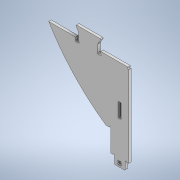
# Autodesk Inventor part: Support A - V2
Saved by Autodesk Inventor 2020 (Build 240168000, 168)
## iProperties
Created: 2020-07-22
Part Number: Support A - V2
Material: Generic
Document SubType Name: Modeling
Designer: Dan Wikman
Density: 1 g/cm^3
Appearance: Default
Author: Dan Wikman
Autodesk Inventor part; units mm, degrees
ref_plane "YZ Plane" through (0, 0, 0) normal (1, 0, 0) x (0, 1, 0)
ref_plane "XZ Plane" through (0, 0, 0) normal (0, 1, 0) x (-1, 0, 0)
ref_plane "XY Plane" through (0, 0, 0) normal (0, 0, 1) x (1, 0, 0)
sketch "Sketch1" plane through (0, 0, 0) normal (0, 0, 1) x (1, 0, 0)
  arc A0 (0, 550) -> (-200, 512.3475) centre (0, 0) ccw construction
  line L0 (-472.3938, -281.6809) -> (-252.3938, -281.6809) construction
  line L1 (-489.0365, 251.6809) -> (-252.3938, 251.6809) construction
  line L2 (-150, 323.3356) -> (-150, 512.3475) construction
  line L3 (-472.3938, 281.6809) -> (-252.3938, 281.6809) construction
  line L4 (-472.3938, -251.6809) -> (-252.3938, -251.6809) construction
  line L5 (-356.435, 15) -> (-576.435, 15) construction
  line L6 (-472.3938, -281.6809) -> (-472.3938, -251.6809) construction
  line L7 (-252.3938, -281.6809) -> (-252.3938, -251.6809) construction
  line L8 (-252.3938, 281.6809) -> (-252.3938, 251.6809) construction
  line L9 (-472.3938, 281.6809) -> (-472.3938, 251.6809) construction
  line L10 (-356.435, 15) -> (-356.435, -15) construction
  line L11 (-356.435, -15) -> (-576.435, -15) construction
  line L12 (-576.435, -15) -> (-576.435, 15) construction
  arc A1 (0, 356.435) -> (-150, 323.3356) centre (0, 0) ccw construction
  arc A2 (-250, -323.3356) -> (-100, -356.435) centre (-100, 0) ccw construction
  arc A3 (-256.5, -512.3475) -> (-260, -512.3475) centre (-258.25, -512.3475) ccw
  line L13 (-278.75, -519.0975) -> (-275, -519.0975)
  line L14 (-278.75, -529.0975) -> (-275, -529.0975)
  line L15 (-275, -519.0975) -> (-275, -529.0975)
  arc A4 (-278.75, -519.0975) -> (-278.75, -522.5975) centre (-278.75, -520.8475) ccw
  arc A5 (-278.75, -525.5975) -> (-278.75, -529.0975) centre (-278.75, -527.3475) ccw
  line L16 (-271.25, -519.0975) -> (-275, -519.0975)
  line L17 (-271.25, -529.0975) -> (-275, -529.0975)
  arc A6 (-271.25, -522.5975) -> (-271.25, -519.0975) centre (-271.25, -520.8475) ccw
  arc A7 (-271.25, -529.0975) -> (-271.25, -525.5975) centre (-271.25, -527.3475) ccw
  line L18 (-356.1192, -15) -> (-549.7954, -15) construction
  line L19 (-252.3938, 251.6809) -> (-489.0365, 251.6809) construction
  arc A8 (-192.6667, 512.3475) -> (-190, 512.3475) centre (-191.3333, 512.3475) ccw construction
  line L20 (-157.3333, 512.3475) -> (-150, 512.3475) construction
  line L21 (-192.6667, 512.3475) -> (-200, 512.3475) construction
  arc A9 (-160, 512.3475) -> (-157.3333, 512.3475) centre (-158.6667, 512.3475) ccw construction
  line L22 (-171.25, 517.8475) -> (-175, 517.8475) construction
  line L23 (-171.25, 520.5142) -> (-171.25, 525.1809) construction
  line L24 (-161.3333, 532.3475) -> (-188.6667, 532.3475) construction
  line L25 (-190, 531.0142) -> (-190, 512.3475) construction
  line L26 (-160, 531.0142) -> (-160, 512.3475) construction
  arc A10 (-160, 531.0142) -> (-161.3333, 532.3475) centre (-161.3333, 531.0142) ccw construction
  arc A11 (-188.6667, 532.3475) -> (-190, 531.0142) centre (-188.6667, 531.0142) ccw construction
  line L27 (-171.25, 527.8475) -> (-175, 527.8475) construction
  line L28 (-175, 532.3475) -> (-175, 535.9358) construction
  line L29 (-175, 517.8475) -> (-175, 527.8475) construction
  arc A12 (-171.25, 517.8475) -> (-171.25, 520.5142) centre (-171.25, 519.1809) ccw construction
  arc A13 (-171.25, 525.1809) -> (-171.25, 527.8475) centre (-171.25, 526.5142) ccw construction
  line L30 (-178.75, 517.8475) -> (-175, 517.8475) construction
  arc A14 (-178.75, 520.5142) -> (-178.75, 517.8475) centre (-178.75, 519.1809) ccw construction
  line L31 (-178.75, 520.5142) -> (-178.75, 525.1809) construction
  arc A15 (-178.75, 527.8475) -> (-178.75, 525.1809) centre (-178.75, 526.5142) ccw construction
  line L32 (-178.75, 527.8475) -> (-175, 527.8475) construction
  arc A16 (-334.9122, -265.623) -> (-335.582, -268.123) centre (-330.582, -268.123) ccw
  line L33 (-328.3782, -254.3059) -> (-334.9122, -265.623)
  arc A17 (-328.3782, -254.3059) -> (-329.8938, -251.6809) centre (-329.8938, -253.4309) ccw
  line L34 (-329.8938, -251.6809) -> (-394.8938, -251.6809)
  line L35 (-362.3938, -251.6809) -> (-362.3938, -293.6041)
  arc A18 (-389.2055, -268.123) -> (-389.8754, -265.623) centre (-394.2055, -268.123) ccw
  arc A19 (-394.8938, -251.6809) -> (-396.4093, -254.3059) centre (-394.8938, -253.4309) ccw
  line L36 (-396.4093, -254.3059) -> (-389.8754, -265.623)
  arc A20 (-389.2055, -291.6809) -> (-389.2055, -288.1809) centre (-389.2055, -289.9309) ccw
  line L37 (-389.2055, -291.6809) -> (-396.7055, -291.6809)
  line L38 (-396.7055, -281.6809) -> (-472.3938, -281.6809)
  line L39 (-328.082, -281.6809) -> (-252.3938, -281.6809)
  arc A21 (-150, 323.3356) -> (-252.3938, -251.6809) centre (0, 0) ccw construction
  arc A22 (-200, 512.3475) -> (-472.3938, -281.6809) centre (0, 0) ccw construction
  line L40 (-271.25, -415.2642) -> (-271.25, -378.7642)
  line L41 (-278.75, -415.2642) -> (-278.75, -378.7642)
  line L42 (-277, -417.0142) -> (-273, -417.0142)
  line L43 (-277, -377.0142) -> (-273, -377.0142)
  arc A23 (-277, -377.0142) -> (-278.75, -378.7642) centre (-277, -378.7642) ccw
  arc A24 (-278.75, -415.2642) -> (-277, -417.0142) centre (-277, -415.2642) ccw
  arc A25 (-273, -417.0142) -> (-271.25, -415.2642) centre (-273, -415.2642) ccw
  arc A26 (-271.25, -378.7642) -> (-273, -377.0142) centre (-273, -378.7642) ccw
  line L44 (-260, -512.3475) -> (-260, -532.5975)
  line L45 (-261.75, -534.3475) -> (-288.25, -534.3475)
  line L46 (-271.25, -522.5975) -> (-271.25, -525.5975)
  line L47 (-278.75, -522.5975) -> (-278.75, -525.5975)
  arc A27 (-290, -532.5975) -> (-288.25, -534.3475) centre (-288.25, -532.5975) ccw
  arc A28 (-261.75, -534.3475) -> (-260, -532.5975) centre (-261.75, -532.5975) ccw
  line L48 (-256.5, -512.3475) -> (-250, -512.3475)
  arc A29 (-396.7055, -288.1809) -> (-396.7055, -291.6809) centre (-396.7055, -289.9309) ccw
  line L49 (-396.7055, -281.6809) -> (-396.7055, -288.1809)
  line L50 (-389.2055, -288.1809) -> (-389.2055, -268.123)
  arc A30 (-335.582, -288.1809) -> (-335.582, -291.6809) centre (-335.582, -289.9309) ccw
  line L51 (-335.582, -291.6809) -> (-328.082, -291.6809)
  arc A31 (-328.082, -291.6809) -> (-328.082, -288.1809) centre (-328.082, -289.9309) ccw
  line L52 (-328.082, -281.6809) -> (-328.082, -288.1809)
  line L53 (-335.582, -288.1809) -> (-335.582, -268.123)
  arc A32 (-252.3938, -283.8475) -> (-252.3938, -287.3475) centre (-252.3938, -285.5975) ccw
  line L54 (-252.3938, -283.8475) -> (-252.3938, -281.6809)
  line L55 (-260, -549.9217) -> (-260, -576.1723)
  line L56 (-160, -561.8521) -> (-260, -561.8521)
  arc A33 (-472.3938, -281.6809) -> (-313.5, -451.9046) centre (0, 0) ccw
  line L57 (-250, -287.3475) -> (-252.3938, -287.3475)
  line L58 (-250, -512.3475) -> (-250, -287.3475)
  arc A34 (-290, -512.3475) -> (-293.5, -512.3475) centre (-291.75, -512.3475) ccw
  line L59 (-293.5, -512.3475) -> (-300, -512.3475)
  line L60 (-300, -512.3475) -> (-300, -451.9046)
  arc A35 (-300, -451.9046) -> (-303.5, -451.9046) centre (-301.75, -451.9046) ccw
  line L61 (-313.5, -451.9046) -> (-303.5, -451.9046)
  line L62 (-290, -532.5975) -> (-290, -512.3475)
  point P0 (0, 512.3475)
  point P1 (0, -512.3475)
  point P2 (-290, -534.3475)
  point P3 (-260, -534.3475)
  point P4 (-59.9119, -534.1417)
  point P5 (-160, 532.3475)
  point P6 (-190, 532.3475)
  point P7 (-389.2055, -259.0142)
  dimension "d13" = 550
  dimension "d17" = 200
  dimension "d18" = 0
  dimension "d54" = 220
  dimension "d56" = 220
  dimension "d57" = 30
  dimension "d59" = 30
  dimension "d62" = 252.3938
  dimension "d73" = 236.6809
  dimension "d74" = 236.6809
  dimension "d75" = 576.435
  dimension "d76" = 472.3938
  dimension "d77" = 472.3938
  dimension "d78" = 30
  dimension "d81" = 220
  dimension "d82" = 252.3938
  dimension "d85" = 356.435
  dimension "d88" = 3.5
  dimension "d89" = 30
  dimension "d90" = 22
  dimension "d103" = 3.75
  dimension "d104" = 3.75
  dimension "d105" = 2.6667
  dimension "d106" = 30
  dimension "d107" = 20
  dimension "d108" = 2.6667
  dimension "d109" = 1.3333
  dimension "d110" = 7.3333
  dimension "d111" = 7.3333
  dimension "d112" = 7.5
  dimension "d113" = 3.75
  dimension "d114" = 3.75
  dimension "d134" = 3.5
  dimension "d135" = 65
  dimension "d136" = 65
  dimension "d137" = 7.3333
  dimension "d138" = 60
  dimension "d139" = 5
  dimension "d140" = 7.5
  dimension "d148" = 1.75
  dimension "d151" = 40
  dimension "d159" = 1.75
  dimension "d160" = 1.75
  dimension "d161" = 1.75
  dimension "d164" = 7.5
  dimension "d170" = 30
  dimension "d171" = 1.75
  dimension "d172" = 10
  dimension "d173" = 3.5
  dimension "d176" = 77.5
  dimension "d180" = 260
  dimension "d182" = 95.3333
  dimension "d184" = 230.6667
  dimension "d185" = 95.3333
  dimension "d186" = 97.0833
  dimension "d187" = 3.5
  constraints: 126 end point, 76 point on circle, 36 centre point, 28 symmetric about line, 16 tangent, 12 vertical, 10 horizontal, 10 perpendicular, 9 point on line, 4 equal radius, 2 collinear, 2 midpoint, 2 parallel, 1 coincident, 10 other
  measures "d13" radius of A0
  measures "d17" distance of point (0, 512.348) A0.end
  measures "d18" horizontal distance of point (0, 0) point (0, 512.348)
  measures "d54" distance of L5.start L5.end
  measures "d56" distance of L0.start L0.end
  measures "d57" distance of L0.end L4.end
  measures "d59" distance between parallel lines of L3 L1
  measures "d62" distance from line of point (0, 0) L7
  measures "d73" distance between parallel lines of L4 L11
  measures "d74" distance between parallel lines of L1 L5
  measures "d75" distance from line of L12 point (0, 0)
  measures "d76" distance from line of point (0, 0) L6
  measures "d77" distance from line of point (0, 0) L9
  measures "d78" distance of L5.start L10.end
  measures "d81" distance between parallel lines of L8 L9
  measures "d82" distance from line of point (0, 0) L8
  measures "d85" distance from line of A0.centre L10
  measures "d88" diameter of A3
  measures "d89" distance of point (-290, -534.348) point (-260, -534.348)
  measures "d90" distance of point (-260, -534.348) L44.start
  measures "d103" distance of L13.start L13.end
  measures "d104" distance of L14.start L14.end
  measures "d105" diameter of A8
  measures "d106" distance of point (-160, 532.348) point (-190, 532.348)
  measures "d107" distance of point (-190, 532.348) L25.end
  measures "d108" diameter of A9
  measures "d109" radius of A10
  measures "d110" distance of L20.start L20.end
  measures "d111" distance of L21.start L21.end
  measures "d112" diameter of L23 L29
  measures "d113" distance of L22.start L22.end
  measures "d114" distance of L27.start L27.end
  measures "d134" diameter of A17
  measures "d135" distance of L34.start L34.end
  measures "d136" distance between centres of A17 A19
  measures "d137" distance from line of point (-389.206, -259.014) L34
  measures "d138" angle of L34 L36
  measures "d139" radius of A18
  measures "d140" distance of L37.start L37.end
  measures "d148" radius of A23
  measures "d151" distance between parallel lines of L42 L43
  measures "d159" radius of A4
  measures "d160" radius of A7
  measures "d161" radius of A27
  measures "d164" distance between parallel lines of L41 L40
  measures "d170" distance between parallel lines of L39 L34
  measures "d171" radius of A20
  measures "d172" distance between parallel lines of L38 L37
  measures "d173" diameter of A32
  measures "d176" horizontal distance of L0.start L34.end
  measures "d180" distance from line of point (0, -512.348) L55
  measures "d182" distance between parallel lines of L42 L48
  measures "d184" distance between parallel lines of L48 L0
  measures "d185" distance between parallel lines of L43 L0
  measures "d186" distance from line of A25.centre L48
  measures "d187" diameter of A35
extrude "Extrusion1" add sketch "Sketch1" along normal blind 7
body "Solid1"
